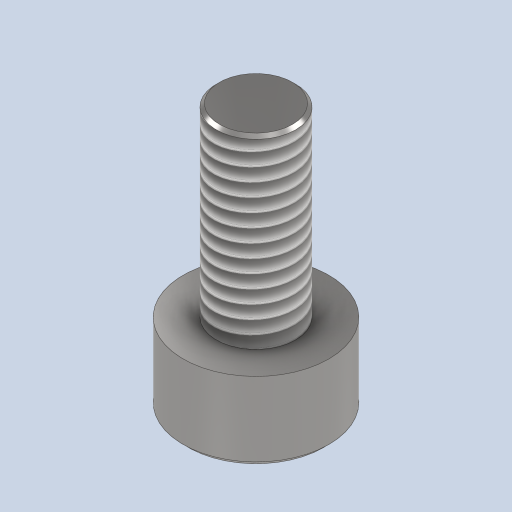
# Autodesk Inventor part: M3_7mm
Saved by Autodesk Inventor 2023 (Build 270158000, 158)
## iProperties
Created: 2024-11-11
Part Number: M3_7mm
Material: ステンレス鋼
Document SubType Name: Modeling
Designer: kiyo
Density: 8 g/cm^3
Appearance: 半つや出し
Author: kiyo
Autodesk Inventor part; units mm, degrees
ref_plane "YZ Plane" through (0, 0, 0) normal (1, 0, 0) x (0, 1, 0)
ref_plane "XZ Plane" through (0, 0, 0) normal (0, 1, 0) x (-1, 0, 0)
ref_plane "XY Plane" through (0, 0, 0) normal (0, 0, 1) x (1, 0, 0)
sketch "スケッチ1" plane through (0, 0, 0) normal (1, 0, 0) x (0, 1, 0)
  line L0 (0, 0) -> (1.5, 0)
  line L1 (1.5, 0) -> (1.5, -7)
  line L2 (1.5, -7) -> (0, -7)
  line L3 (0, -7) -> (0, 0)
  line L4 (0, -7) -> (2.75, -7)
  line L5 (2.75, -7) -> (2.75, -10)
  line L6 (2.75, -10) -> (0, -10)
  line L7 (0, -10) -> (0, -7)
  line L8 (2.75, -9.8) -> (2.55, -10)
  line L9 (1.5, -0.12) -> (1.38, 0)
  point P0 (2.75, -8.5)
  dimension "d0" = 45
  dimension "d1" = 2.75
  dimension "d2" = 3
  dimension "d3" = 7
  dimension "d7" = 1.5
  dimension "d10" = 45
  dimension "d11" = 0.12
  dimension "d12" = 0.2
  constraints: 20 end point, 4 parallel, 4 point on line, 2 horizontal, 2 perpendicular, 1 midpoint
  measures "d0" angle of L8 L5
  measures "d1" distance from line of L7 point (2.75, -8.5)
  measures "d2" distance of L4.end L5.end
  measures "d3" distance of L0.end L1.end
  measures "d7" distance between parallel lines of L3 L1
  measures "d10" angle of L9 L1
  measures "d11" distance from line of L0 L9.start
  measures "d12" distance from line of L5 L8.end
revolve "回転1" add sketch "スケッチ1" angle 360 about axis through (0, 0, -7) along (0, 0, 1) contours L0 L9 L1 L2 L3 | L2 L4 L5 L8 L6 L7
thread "ねじ2" size "M3x0.5" class "6g" standard "ANSI Metric M Profile" length 30
